Autodesk Fusion 360 part; units mm, degrees
(part 8 of 8)
  spline S32 degree 5 poles (-90.0942, -119.2775) (-90.131, -119.331) (-90.2033, -119.4387) (-90.3076, -119.6028) (-90.4386, -119.8264) (-90.5914, -120.1126) (-90.7364, -120.4035) (-90.8766, -120.6973) (-91.0142, -120.9926) (-91.1501, -121.289) (-91.284, -121.5864) (-91.4155, -121.8852) (-91.5436, -122.1859) (-91.6678, -122.4887) (-91.7881, -122.7937) (-91.9048, -123.1006) (-92.0185, -123.4092) (-92.1295, -123.7191) (-92.2384, -124.0301) (-92.3451, -124.3422) (-92.4496, -124.6553) (-92.5518, -124.9696) (-92.6517, -125.285) (-92.7491, -125.6017) (-92.844, -125.9195) (-92.9366, -126.2385) (-93.027, -126.5585) (-93.1153, -126.8794) (-93.2015, -127.2013) (-93.2857, -127.5241) (-93.368, -127.8478) (-93.4482, -128.1724) (-93.5264, -128.4978) (-93.6027, -128.8241) (-93.6769, -129.1513) (-93.7493, -129.4793) (-93.8197, -129.808) (-93.8882, -130.1376) (-93.9549, -130.4679) (-94.0198, -130.7989) (-94.0829, -131.1307) (-94.1441, -131.4631) (-94.2036, -131.7963) (-94.2613, -132.1301) (-94.3172, -132.4646) (-94.3714, -132.7998) (-94.4239, -133.1356) (-94.4747, -133.4721) (-94.5237, -133.8091) (-94.5711, -134.1468) (-94.6168, -134.4851) (-94.6609, -134.8239) (-94.7033, -135.1634) (-94.744, -135.5033) (-94.7831, -135.8439) (-94.8206, -136.185) (-94.8565, -136.5266) (-94.8908, -136.8687) (-94.9235, -137.2114) (-94.9546, -137.5545) (-94.9842, -137.8982) (-95.0122, -138.2423) (-95.0386, -138.5869) (-95.0635, -138.932) (-95.0869, -139.2775) (-95.1087, -139.6235) (-95.129, -139.97) (-95.1478, -140.3168) (-95.1651, -140.6641) (-95.1808, -141.0118) (-95.1951, -141.36) (-95.2054, -141.6388) (-95.2124, -141.8481) (-95.2168, -141.9877) (-95.2189, -142.0576) knots 0 0 0 0 0 0 0.01428571 0.02857143 0.04285714 0.05714286 0.07142857 0.08571429 0.1 0.11428571 0.12857143 0.14285714 0.15714286 0.17142857 0.18571429 0.2 0.21428571 0.22857143 0.24285714 0.25714286 0.27142857 0.28571429 0.3 0.31428571 0.32857143 0.34285714 0.35714286 0.37142857 0.38571429 0.4 0.41428571 0.42857143 0.44285714 0.45714286 0.47142857 0.48571429 0.5 0.51428571 0.52857143 0.54285714 0.55714286 0.57142857 0.58571429 0.6 0.61428571 0.62857143 0.64285714 0.65714286 0.67142857 0.68571429 0.7 0.71428571 0.72857143 0.74285714 0.75714286 0.77142857 0.78571429 0.8 0.81428571 0.82857143 0.84285714 0.85714286 0.87142857 0.88571429 0.9 0.91428571 0.92857143 0.94285714 0.95714286 0.97142857 0.98571429 1 1 1 1 1 1
  arc A66 (-95.2189, -142.0576) -> (-87.3499, -146.6007) centre (-8.7656, -1.4025) ccw
  spline S33 degree 5 poles (-87.3499, -146.6007) (-87.2904, -146.564) (-87.1717, -146.4904) (-86.9939, -146.3797) (-86.7576, -146.2314) (-86.4632, -146.0449) (-86.17, -145.8574) (-85.8779, -145.6688) (-85.5869, -145.4791) (-85.297, -145.2883) (-85.0083, -145.0964) (-84.7207, -144.9034) (-84.4343, -144.7093) (-84.1491, -144.5141) (-83.865, -144.3178) (-83.5822, -144.1204) (-83.3006, -143.9219) (-83.0202, -143.7222) (-82.7411, -143.5214) (-82.4632, -143.3196) (-82.1865, -143.1165) (-81.9112, -142.9124) (-81.6371, -142.7071) (-81.3644, -142.5007) (-81.0929, -142.2931) (-80.8228, -142.0844) (-80.5541, -141.8745) (-80.2867, -141.6635) (-80.0207, -141.4513) (-79.7561, -141.238) (-79.4929, -141.0235) (-79.2312, -140.8077) (-78.9709, -140.5908) (-78.7122, -140.3728) (-78.4549, -140.1535) (-78.1991, -139.933) (-77.9449, -139.7113) (-77.6922, -139.4884) (-77.441, -139.2642) (-77.1915, -139.0389) (-76.9437, -138.8122) (-76.6975, -138.5844) (-76.453, -138.3552) (-76.2103, -138.1247) (-75.9693, -137.8929) (-75.7301, -137.6599) (-75.4927, -137.4256) (-75.257, -137.1899) (-75.0232, -136.953) (-74.7912, -136.7147) (-74.5613, -136.475) (-74.3336, -136.2339) (-74.108, -135.9912) (-73.8848, -135.747) (-73.6637, -135.5014) (-73.4448, -135.2543) (-73.2279, -135.0058) (-73.0129, -134.7561) (-72.8001, -134.5049) (-72.5897, -134.2522) (-72.3823, -133.9976) (-72.1783, -133.741) (-71.9781, -133.482) (-71.7818, -133.2207) (-71.5887, -132.9575) (-71.3981, -132.6928) (-71.2094, -132.4269) (-71.0224, -132.1601) (-70.8381, -131.8918) (-70.6587, -131.6207) (-70.4873, -131.3453) (-70.3591, -131.1201) (-70.2691, -130.9477) (-70.212, -130.8313) (-70.1841, -130.7726) knots -1 -1 -1 -1 -1 -1 -0.98571429 -0.97142857 -0.95714286 -0.94285714 -0.92857143 -0.91428571 -0.9 -0.88571429 -0.87142857 -0.85714286 -0.84285714 -0.82857143 -0.81428571 -0.8 -0.78571429 -0.77142857 -0.75714286 -0.74285714 -0.72857143 -0.71428571 -0.7 -0.68571429 -0.67142857 -0.65714286 -0.64285714 -0.62857143 -0.61428571 -0.6 -0.58571429 -0.57142857 -0.55714286 -0.54285714 -0.52857143 -0.51428571 -0.5 -0.48571429 -0.47142857 -0.45714286 -0.44285714 -0.42857143 -0.41428571 -0.4 -0.38571429 -0.37142857 -0.35714286 -0.34285714 -0.32857143 -0.31428571 -0.3 -0.28571429 -0.27142857 -0.25714286 -0.24285714 -0.22857143 -0.21428571 -0.2 -0.18571429 -0.17142857 -0.15714286 -0.14285714 -0.12857143 -0.11428571 -0.1 -0.08571429 -0.07142857 -0.05714286 -0.04285714 -0.02857143 -0.01428571 0 0 0 0 0 0
  line L33 (-70.1841, -130.7726) -> (-68.2443, -126.6881)
  arc A67 (-66.146, -125.9273) -> (-68.2443, -126.6881) centre (-66.8103, -127.3691) ccw
  arc A68 (-66.146, -125.9273) -> (-56.2439, -130.0289) centre (-8.7656, -1.4025) ccw
  arc A69 (-55.2981, -132.0506) -> (-56.2439, -130.0289) centre (-56.7937, -131.5181) ccw
  line L34 (-55.2981, -132.0506) -> (-56.8147, -136.3104)
  spline S34 degree 5 poles (-56.8147, -136.3104) (-56.8364, -136.3716) (-56.8784, -136.4943) (-56.9366, -136.6798) (-57.0053, -136.9297) (-57.0788, -137.2457) (-57.1436, -137.5642) (-57.203, -137.8843) (-57.2595, -138.2052) (-57.314, -138.5266) (-57.3664, -138.8486) (-57.416, -139.1712) (-57.4619, -139.4948) (-57.5035, -139.8195) (-57.5408, -140.1452) (-57.5741, -140.4719) (-57.604, -140.7993) (-57.6311, -141.1274) (-57.6557, -141.456) (-57.678, -141.7851) (-57.6979, -142.1146) (-57.7154, -142.4446) (-57.7302, -142.7751) (-57.7423, -143.1062) (-57.7517, -143.4378) (-57.7586, -143.7698) (-57.7631, -144.1023) (-57.7653, -144.4352) (-57.7653, -144.7685) (-57.7631, -145.1021) (-57.7588, -145.436) (-57.7523, -145.7703) (-57.7436, -146.1049) (-57.7328, -146.4398) (-57.7198, -146.775) (-57.7048, -147.1105) (-57.6877, -147.4463) (-57.6686, -147.7824) (-57.6476, -148.1187) (-57.6246, -148.4552) (-57.5996, -148.792) (-57.5728, -149.129) (-57.544, -149.4662) (-57.5133, -149.8036) (-57.4808, -150.1412) (-57.4464, -150.479) (-57.4101, -150.8169) (-57.3721, -151.1551) (-57.3322, -151.4933) (-57.2906, -151.8318) (-57.2472, -152.1703) (-57.202, -152.509) (-57.1551, -152.8479) (-57.1065, -153.1868) (-57.0562, -153.5259) (-57.0041, -153.865) (-56.9504, -154.2043) (-56.8949, -154.5437) (-56.8378, -154.8831) (-56.7791, -155.2226) (-56.7187, -155.5622) (-56.6567, -155.9019) (-56.593, -156.2416) (-56.5277, -156.5813) (-56.4609, -156.9211) (-56.3924, -157.261) (-56.3223, -157.6009) (-56.2507, -157.9408) (-56.1775, -158.2807) (-56.1028, -158.6207) (-56.0265, -158.9606) (-55.9642, -159.2326) (-55.9168, -159.4366) (-55.8849, -159.5726) (-55.8688, -159.6406) knots 0 0 0 0 0 0 0.01428571 0.02857143 0.04285714 0.05714286 0.07142857 0.08571429 0.1 0.11428571 0.12857143 0.14285714 0.15714286 0.17142857 0.18571429 0.2 0.21428571 0.22857143 0.24285714 0.25714286 0.27142857 0.28571429 0.3 0.31428571 0.32857143 0.34285714 0.35714286 0.37142857 0.38571429 0.4 0.41428571 0.42857143 0.44285714 0.45714286 0.47142857 0.48571429 0.5 0.51428571 0.52857143 0.54285714 0.55714286 0.57142857 0.58571429 0.6 0.61428571 0.62857143 0.64285714 0.65714286 0.67142857 0.68571429 0.7 0.71428571 0.72857143 0.74285714 0.75714286 0.77142857 0.78571429 0.8 0.81428571 0.82857143 0.84285714 0.85714286 0.87142857 0.88571429 0.9 0.91428571 0.92857143 0.94285714 0.95714286 0.97142857 0.98571429 1 1 1 1 1 1
  arc A70 (-55.8688, -159.6406) -> (-47.0921, -161.9923) centre (-8.7656, -1.4025) ccw
  spline S35 degree 5 poles (-47.0921, -161.9923) (-47.0442, -161.9414) (-46.9486, -161.8396) (-46.8055, -161.6867) (-46.6156, -161.4823) (-46.3795, -161.226) (-46.1448, -160.969) (-45.9115, -160.7112) (-45.6795, -160.4526) (-45.4489, -160.1933) (-45.2197, -159.9332) (-44.9918, -159.6724) (-44.7654, -159.4108) (-44.5404, -159.1484) (-44.3169, -158.8853) (-44.0948, -158.6214) (-43.8742, -158.3567) (-43.655, -158.0913) (-43.4373, -157.8251) (-43.2211, -157.5582) (-43.0065, -157.2905) (-42.7933, -157.022) (-42.5817, -156.7528) (-42.3717, -156.4828) (-42.1633, -156.2121) (-41.9564, -155.9406) (-41.7511, -155.6683) (-41.5475, -155.3952) (-41.3455, -155.1215) (-41.1451, -154.8469) (-40.9464, -154.5716) (-40.7494, -154.2955) (-40.5542, -154.0186) (-40.3606, -153.741) (-40.1689, -153.4626) (-39.9789, -153.1834) (-39.7907, -152.9034) (-39.6043, -152.6227) (-39.4197, -152.3412) (-39.2371, -152.0589) (-39.0563, -151.7759) (-38.8775, -151.4921) (-38.7006, -151.2074) (-38.5258, -150.922) (-38.3531, -150.6357) (-38.1823, -150.3487) (-38.0136, -150.0609) (-37.847, -149.7723) (-37.6825, -149.4829) (-37.5201, -149.1928) (-37.36, -148.9017) (-37.2024, -148.6098) (-37.0474, -148.3171) (-36.8949, -148.0234) (-36.745, -147.7289) (-36.5975, -147.4336) (-36.4523, -147.1375) (-36.3093, -146.8406) (-36.1687, -146.5429) (-36.0309, -146.2443) (-35.8964, -145.9448) (-35.7659, -145.6441) (-35.6395, -145.3421) (-35.5175, -145.0389) (-35.3991, -144.7347) (-35.2835, -144.4296) (-35.17, -144.124) (-35.0585, -143.8179) (-34.9499, -143.511) (-34.8468, -143.2028) (-34.7525, -142.8924) (-34.687, -142.6416) (-34.6446, -142.4518) (-34.6196, -142.3246) (-34.6079, -142.2607) knots -1 -1 -1 -1 -1 -1 -0.98571429 -0.97142857 -0.95714286 -0.94285714 -0.92857143 -0.91428571 -0.9 -0.88571429 -0.87142857 -0.85714286 -0.84285714 -0.82857143 -0.81428571 -0.8 -0.78571429 -0.77142857 -0.75714286 -0.74285714 -0.72857143 -0.71428571 -0.7 -0.68571429 -0.67142857 -0.65714286 -0.64285714 -0.62857143 -0.61428571 -0.6 -0.58571429 -0.57142857 -0.55714286 -0.54285714 -0.52857143 -0.51428571 -0.5 -0.48571429 -0.47142857 -0.45714286 -0.44285714 -0.42857143 -0.41428571 -0.4 -0.38571429 -0.37142857 -0.35714286 -0.34285714 -0.32857143 -0.31428571 -0.3 -0.28571429 -0.27142857 -0.25714286 -0.24285714 -0.22857143 -0.21428571 -0.2 -0.18571429 -0.17142857 -0.15714286 -0.14285714 -0.12857143 -0.11428571 -0.1 -0.08571429 -0.07142857 -0.05714286 -0.04285714 -0.02857143 -0.01428571 0 0 0 0 0 0
  line L35 (-34.6079, -142.2607) -> (-33.7913, -137.8133)
  arc A71 (-31.9614, -136.5354) -> (-33.7913, -137.8133) centre (-32.2299, -138.1) ccw
  arc A72 (-31.9614, -136.5354) -> (-21.3352, -137.9343) centre (-8.7656, -1.4025) ccw
  arc A73 (-19.8983, -139.6424) -> (-21.3352, -137.9343) centre (-21.4807, -139.5151) ccw
  line L36 (-19.8983, -139.6424) -> (-20.2607, -144.1496)
  spline S36 degree 5 poles (-20.2607, -144.1496) (-20.2659, -144.2143) (-20.2747, -144.3437) (-20.2829, -144.5379) (-20.2845, -144.7971) (-20.2738, -145.1213) (-20.2539, -145.4457) (-20.2284, -145.7703) (-20.1999, -146.0949) (-20.1694, -146.4194) (-20.1367, -146.744) (-20.1011, -147.0685) (-20.0617, -147.3929) (-20.0179, -147.7173) (-19.9696, -148.0416) (-19.9172, -148.3658) (-19.8613, -148.6898) (-19.8026, -149.0137) (-19.7413, -149.3375) (-19.6777, -149.6611) (-19.6116, -149.9846) (-19.5431, -150.3078) (-19.4718, -150.631) (-19.3978, -150.9539) (-19.3211, -151.2766) (-19.2419, -151.5991) (-19.1601, -151.9214) (-19.0761, -152.2436) (-18.9898, -152.5654) (-18.9014, -152.8871) (-18.8107, -153.2085) (-18.718, -153.5297) (-18.623, -153.8507) (-18.5259, -154.1714) (-18.4266, -154.4918) (-18.3252, -154.812) (-18.2218, -155.132) (-18.1164, -155.4516) (-18.009, -155.771) (-17.8997, -156.0902) (-17.7884, -156.409) (-17.6753, -156.7275) (-17.5602, -157.0458) (-17.4432, -157.3638) (-17.3244, -157.6815) (-17.2038, -157.9988) (-17.0813, -158.3159) (-16.957, -158.6326) (-16.831, -158.9491) (-16.7032, -159.2652) (-16.5736, -159.581) (-16.4424, -159.8965) (-16.3094, -160.2116) (-16.1747, -160.5264) (-16.0383, -160.8409) (-15.9002, -161.155) (-15.7605, -161.4688) (-15.6191, -161.7823) (-15.4761, -162.0954) (-15.3315, -162.4081) (-15.1853, -162.7205) (-15.0374, -163.0325) (-14.888, -163.3442) (-14.737, -163.6555) (-14.5845, -163.9664) (-14.4304, -164.277) (-14.2748, -164.5871) (-14.1176, -164.8969) (-13.9589, -165.2063) (-13.7987, -165.5153) (-13.637, -165.824) (-13.5065, -166.0706) (-13.4079, -166.2553) (-13.3419, -166.3784) (-13.3088, -166.44) knots 0 0 0 0 0 0 0.01428571 0.02857143 0.04285714 0.05714286 0.07142857 0.08571429 0.1 0.11428571 0.12857143 0.14285714 0.15714286 0.17142857 0.18571429 0.2 0.21428571 0.22857143 0.24285714 0.25714286 0.27142857 0.28571429 0.3 0.31428571 0.32857143 0.34285714 0.35714286 0.37142857 0.38571429 0.4 0.41428571 0.42857143 0.44285714 0.45714286 0.47142857 0.48571429 0.5 0.51428571 0.52857143 0.54285714 0.55714286 0.57142857 0.58571429 0.6 0.61428571 0.62857143 0.64285714 0.65714286 0.67142857 0.68571429 0.7 0.71428571 0.72857143 0.74285714 0.75714286 0.77142857 0.78571429 0.8 0.81428571 0.82857143 0.84285714 0.85714286 0.87142857 0.88571429 0.9 0.91428571 0.92857143 0.94285714 0.95714286 0.97142857 0.98571429 1 1 1 1 1 1
  arc A74 (-13.3088, -166.44) -> (-4.2224, -166.44) centre (-8.7656, -1.4025) ccw
  spline S37 degree 5 poles (-4.2224, -166.44) (-4.1894, -166.3784) (-4.1233, -166.2553) (-4.0248, -166.0706) (-3.8942, -165.824) (-3.7325, -165.5153) (-3.5723, -165.2063) (-3.4136, -164.8969) (-3.2565, -164.5871) (-3.1008, -164.277) (-2.9468, -163.9664) (-2.7942, -163.6555) (-2.6432, -163.3442) (-2.4938, -163.0325) (-2.346, -162.7205) (-2.1997, -162.4081) (-2.0551, -162.0954) (-1.9121, -161.7823) (-1.7708, -161.4688) (-1.631, -161.155) (-1.493, -160.8409) (-1.3566, -160.5264) (-1.2219, -160.2116) (-1.0889, -159.8965) (-0.9576, -159.581) (-0.828, -159.2652) (-0.7002, -158.9491) (-0.5742, -158.6326) (-0.4499, -158.3159) (-0.3275, -157.9988) (-0.2068, -157.6815) (-0.088, -157.3638) (0.029, -157.0458) (0.144, -156.7275) (0.2572, -156.409) (0.3685, -156.0902) (0.4778, -155.771) (0.5852, -155.4516) (0.6906, -155.132) (0.794, -154.812) (0.8953, -154.4918) (0.9946, -154.1714) (1.0917, -153.8507) (1.1867, -153.5297) (1.2795, -153.2085) (1.3701, -152.8871) (1.4586, -152.5654) (1.5449, -152.2436) (1.6289, -151.9214) (1.7106, -151.5991) (1.7899, -151.2766) (1.8666, -150.9539) (1.9406, -150.631) (2.0118, -150.3078) (2.0804, -149.9846) (2.1464, -149.6611) (2.2101, -149.3375) (2.2713, -149.0137) (2.3301, -148.6898) (2.386, -148.3658) (2.4383, -148.0416) (2.4866, -147.7173) (2.5305, -147.3929) (2.5699, -147.0685) (2.6055, -146.744) (2.6382, -146.4194) (2.6687, -146.0949) (2.6972, -145.7703) (2.7227, -145.4457) (2.7425, -145.1213) (2.7533, -144.7971) (2.7516, -144.5379) (2.7434, -144.3437) (2.7347, -144.2143) (2.7295, -144.1496) knots -1 -1 -1 -1 -1 -1 -0.98571429 -0.97142857 -0.95714286 -0.94285714 -0.92857143 -0.91428571 -0.9 -0.88571429 -0.87142857 -0.85714286 -0.84285714 -0.82857143 -0.81428571 -0.8 -0.78571429 -0.77142857 -0.75714286 -0.74285714 -0.72857143 -0.71428571 -0.7 -0.68571429 -0.67142857 -0.65714286 -0.64285714 -0.62857143 -0.61428571 -0.6 -0.58571429 -0.57142857 -0.55714286 -0.54285714 -0.52857143 -0.51428571 -0.5 -0.48571429 -0.47142857 -0.45714286 -0.44285714 -0.42857143 -0.41428571 -0.4 -0.38571429 -0.37142857 -0.35714286 -0.34285714 -0.32857143 -0.31428571 -0.3 -0.28571429 -0.27142857 -0.25714286 -0.24285714 -0.22857143 -0.21428571 -0.2 -0.18571429 -0.17142857 -0.15714286 -0.14285714 -0.12857143 -0.11428571 -0.1 -0.08571429 -0.07142857 -0.05714286 -0.04285714 -0.02857143 -0.01428571 0 0 0 0 0 0
  line L37 (2.7295, -144.1496) -> (2.3671, -139.6424)
  arc A75 (3.804, -137.9343) -> (2.3671, -139.6424) centre (3.9495, -139.5151) ccw
  arc A76 (3.804, -137.9343) -> (14.4301, -136.5354) centre (-8.7656, -1.4025) ccw
  arc A77 (16.2601, -137.8133) -> (14.4301, -136.5354) centre (14.6987, -138.1) ccw
  line L38 (16.2601, -137.8133) -> (17.0766, -142.2607)
  spline S38 degree 5 poles (17.0766, -142.2607) (17.0884, -142.3246) (17.1134, -142.4518) (17.1557, -142.6416) (17.2212, -142.8924) (17.3155, -143.2028) (17.4187, -143.511) (17.5273, -143.8179) (17.6388, -144.124) (17.7523, -144.4296) (17.8679, -144.7347) (17.9862, -145.0389) (18.1083, -145.3421) (18.2346, -145.6441) (18.3652, -145.9448) (18.4997, -146.2443) (18.6375, -146.5429) (18.7781, -146.8406) (18.9211, -147.1375) (19.0663, -147.4336) (19.2138, -147.7289) (19.3637, -148.0234) (19.5162, -148.3171) (19.6712, -148.6098) (19.8288, -148.9017) (19.9889, -149.1928) (20.1512, -149.4829) (20.3158, -149.7723) (20.4824, -150.0609) (20.6511, -150.3487) (20.8218, -150.6357) (20.9946, -150.922) (21.1694, -151.2074) (21.3462, -151.4921) (21.525, -151.7759) (21.7058, -152.0589) (21.8885, -152.3412) (22.0731, -152.6227) (22.2594, -152.9034) (22.4476, -153.1834) (22.6376, -153.4626) (22.8294, -153.741) (23.0229, -154.0186) (23.2182, -154.2955) (23.4152, -154.5716) (23.6139, -154.8469) (23.8142, -155.1215) (24.0162, -155.3952) (24.2199, -155.6683) (24.4251, -155.9406) (24.632, -156.2121) (24.8405, -156.4828) (25.0505, -156.7528) (25.2621, -157.022) (25.4752, -157.2905) (25.6899, -157.5582) (25.9061, -157.8251) (26.1238, -158.0913) (26.3429, -158.3567) (26.5636, -158.6214) (26.7857, -158.8853) (27.0092, -159.1484) (27.2342, -159.4108) (27.4606, -159.6724) (27.6884, -159.9332) (27.9176, -160.1933) (28.1483, -160.4526) (28.3802, -160.7112) (28.6136, -160.969) (28.8483, -161.226) (29.0844, -161.4823) (29.2743, -161.6867) (29.4173, -161.8396) (29.513, -161.9414) (29.5609, -161.9923) knots 0 0 0 0 0 0 0.01428571 0.02857143 0.04285714 0.05714286 0.07142857 0.08571429 0.1 0.11428571 0.12857143 0.14285714 0.15714286 0.17142857 0.18571429 0.2 0.21428571 0.22857143 0.24285714 0.25714286 0.27142857 0.28571429 0.3 0.31428571 0.32857143 0.34285714 0.35714286 0.37142857 0.38571429 0.4 0.41428571 0.42857143 0.44285714 0.45714286 0.47142857 0.48571429 0.5 0.51428571 0.52857143 0.54285714 0.55714286 0.57142857 0.58571429 0.6 0.61428571 0.62857143 0.64285714 0.65714286 0.67142857 0.68571429 0.7 0.71428571 0.72857143 0.74285714 0.75714286 0.77142857 0.78571429 0.8 0.81428571 0.82857143 0.84285714 0.85714286 0.87142857 0.88571429 0.9 0.91428571 0.92857143 0.94285714 0.95714286 0.97142857 0.98571429 1 1 1 1 1 1
  arc A78 (29.5609, -161.9923) -> (38.3376, -159.6406) centre (-8.7656, -1.4025) ccw
  spline S39 degree 5 poles (38.3376, -159.6406) (38.3536, -159.5726) (38.3855, -159.4366) (38.4329, -159.2326) (38.4952, -158.9606) (38.5715, -158.6207) (38.6463, -158.2807) (38.7195, -157.9408) (38.7911, -157.6009) (38.8611, -157.261) (38.9296, -156.9211) (38.9965, -156.5813) (39.0618, -156.2416) (39.1254, -155.9019) (39.1875, -155.5622) (39.2478, -155.2226) (39.3066, -154.8831) (39.3637, -154.5437) (39.4191, -154.2043) (39.4729, -153.865) (39.5249, -153.5259) (39.5753, -153.1868) (39.6239, -152.8479) (39.6708, -152.509) (39.716, -152.1703) (39.7594, -151.8318) (39.801, -151.4933) (39.8408, -151.1551) (39.8789, -150.8169) (39.9151, -150.479) (39.9495, -150.1412) (39.9821, -149.8036) (40.0127, -149.4662) (40.0415, -149.129) (40.0684, -148.792) (40.0933, -148.4552) (40.1163, -148.1187) (40.1374, -147.7824) (40.1565, -147.4463) (40.1736, -147.1105) (40.1886, -146.775) (40.2015, -146.4398) (40.2124, -146.1049) (40.221, -145.7703) (40.2275, -145.436) (40.2319, -145.1021) (40.2341, -144.7685) (40.2341, -144.4352) (40.2319, -144.1023) (40.2274, -143.7698) (40.2205, -143.4378) (40.211, -143.1062) (40.1989, -142.7751) (40.1841, -142.4446) (40.1667, -142.1146) (40.1468, -141.7851) (40.1245, -141.456) (40.0999, -141.1274) (40.0728, -140.7993) (40.0429, -140.4719) (40.0095, -140.1452) (39.9723, -139.8195) (39.9307, -139.4948) (39.8848, -139.1712) (39.8352, -138.8486) (39.7827, -138.5266) (39.7282, -138.2052) (39.6717, -137.8843) (39.6123, -137.5642) (39.5476, -137.2457) (39.474, -136.9297) (39.4054, -136.6798) (39.3472, -136.4943) (39.3052, -136.3716) (39.2834, -136.3104) knots -1 -1 -1 -1 -1 -1 -0.98571429 -0.97142857 -0.95714286 -0.94285714 -0.92857143 -0.91428571 -0.9 -0.88571429 -0.87142857 -0.85714286 -0.84285714 -0.82857143 -0.81428571 -0.8 -0.78571429 -0.77142857 -0.75714286 -0.74285714 -0.72857143 -0.71428571 -0.7 -0.68571429 -0.67142857 -0.65714286 -0.64285714 -0.62857143 -0.61428571 -0.6 -0.58571429 -0.57142857 -0.55714286 -0.54285714 -0.52857143 -0.51428571 -0.5 -0.48571429 -0.47142857 -0.45714286 -0.44285714 -0.42857143 -0.41428571 -0.4 -0.38571429 -0.37142857 -0.35714286 -0.34285714 -0.32857143 -0.31428571 -0.3 -0.28571429 -0.27142857 -0.25714286 -0.24285714 -0.22857143 -0.21428571 -0.2 -0.18571429 -0.17142857 -0.15714286 -0.14285714 -0.12857143 -0.11428571 -0.1 -0.08571429 -0.07142857 -0.05714286 -0.04285714 -0.02857143 -0.01428571 0 0 0 0 0 0
  line L39 (39.2834, -136.3104) -> (37.7669, -132.0506)
  arc A79 (38.7127, -130.0289) -> (37.7669, -132.0506) centre (39.2624, -131.5181) ccw
  arc A80 (38.7127, -130.0289) -> (48.6147, -125.9273) centre (-8.7656, -1.4025) ccw
  arc A81 (50.7131, -126.6881) -> (48.6147, -125.9273) centre (49.2791, -127.3691) ccw
  line L40 (50.7131, -126.6881) -> (52.6529, -130.7726)
  spline S40 degree 5 poles (52.6529, -130.7726) (52.6807, -130.8313) (52.7378, -130.9477) (52.8278, -131.1201) (52.956, -131.3453) (53.1274, -131.6207) (53.3069, -131.8918) (53.4912, -132.1601) (53.6781, -132.4269) (53.8669, -132.6928) (54.0575, -132.9575) (54.2505, -133.2207) (54.4469, -133.482) (54.6471, -133.741) (54.851, -133.9976) (55.0585, -134.2522) (55.2689, -134.5049) (55.4817, -134.7561) (55.6966, -135.0058) (55.9136, -135.2543) (56.1325, -135.5014) (56.3535, -135.747) (56.5768, -135.9912) (56.8023, -136.2339) (57.0301, -136.475) (57.26, -136.7147) (57.4919, -136.953) (57.7258, -137.1899) (57.9614, -137.4256) (58.1989, -137.6599) (58.4381, -137.8929) (58.679, -138.1247) (58.9217, -138.3552) (59.1662, -138.5844) (59.4124, -138.8122) (59.6603, -139.0389) (59.9098, -139.2642) (60.1609, -139.4884) (60.4136, -139.7113) (60.6679, -139.933) (60.9236, -140.1535) (61.1809, -140.3728) (61.4397, -140.5908) (61.7, -140.8077) (61.9617, -141.0235) (62.2249, -141.238) (62.4895, -141.4513) (62.7555, -141.6635) (63.0228, -141.8745) (63.2916, -142.0844) (63.5617, -142.2931) (63.8331, -142.5007) (64.1059, -142.7071) (64.3799, -142.9124) (64.6553, -143.1165) (64.9319, -143.3196) (65.2098, -143.5214) (65.489, -143.7222) (65.7694, -143.9219) (66.051, -144.1204) (66.3338, -144.3178) (66.6178, -144.5141) (66.9031, -144.7093) (67.1895, -144.9034) (67.477, -145.0964) (67.7658, -145.2883) (68.0556, -145.4791) (68.3466, -145.6688) (68.6388, -145.8574) (68.932, -146.0449) (69.2263, -146.2314) (69.4627, -146.3797) (69.6405, -146.4904) (69.7592, -146.564) (69.8186, -146.6007) knots 0 0 0 0 0 0 0.01428571 0.02857143 0.04285714 0.05714286 0.07142857 0.08571429 0.1 0.11428571 0.12857143 0.14285714 0.15714286 0.17142857 0.18571429 0.2 0.21428571 0.22857143 0.24285714 0.25714286 0.27142857 0.28571429 0.3 0.31428571 0.32857143 0.34285714 0.35714286 0.37142857 0.38571429 0.4 0.41428571 0.42857143 0.44285714 0.45714286 0.47142857 0.48571429 0.5 0.51428571 0.52857143 0.54285714 0.55714286 0.57142857 0.58571429 0.6 0.61428571 0.62857143 0.64285714 0.65714286 0.67142857 0.68571429 0.7 0.71428571 0.72857143 0.74285714 0.75714286 0.77142857 0.78571429 0.8 0.81428571 0.82857143 0.84285714 0.85714286 0.87142857 0.88571429 0.9 0.91428571 0.92857143 0.94285714 0.95714286 0.97142857 0.98571429 1 1 1 1 1 1
  arc A82 (69.8186, -146.6007) -> (77.6876, -142.0576) centre (-8.7656, -1.4025) ccw
  spline S41 degree 5 poles (77.6876, -142.0576) (77.6855, -141.9877) (77.6811, -141.8481) (77.6741, -141.6388) (77.6639, -141.36) (77.6496, -141.0118) (77.6338, -140.6641) (77.6165, -140.3168) (77.5977, -139.97) (77.5774, -139.6235) (77.5556, -139.2775) (77.5323, -138.932) (77.5074, -138.5869) (77.4809, -138.2423) (77.453, -137.8982) (77.4234, -137.5545) (77.3923, -137.2114) (77.3596, -136.8687) (77.3253, -136.5266) (77.2894, -136.185) (77.2519, -135.8439) (77.2128, -135.5033) (77.172, -135.1634) (77.1296, -134.8239) (77.0856, -134.4851) (77.0399, -134.1468) (76.9925, -133.8091) (76.9434, -133.4721) (76.8927, -133.1356) (76.8402, -132.7998) (76.786, -132.4646) (76.7301, -132.1301) (76.6724, -131.7963) (76.6129, -131.4631) (76.5516, -131.1307) (76.4886, -130.7989) (76.4237, -130.4679) (76.357, -130.1376) (76.2884, -129.808) (76.218, -129.4793) (76.1457, -129.1513) (76.0714, -128.8241) (75.9952, -128.4978) (75.917, -128.1724) (75.8367, -127.8478) (75.7545, -127.5241) (75.6703, -127.2013) (75.584, -126.8794) (75.4958, -126.5585) (75.4054, -126.2385) (75.3128, -125.9195) (75.2178, -125.6017) (75.1204, -125.285) (75.0206, -124.9696) (74.9183, -124.6553) (74.8138, -124.3422) (74.7071, -124.0301) (74.5983, -123.7191) (74.4872, -123.4092) (74.3736, -123.1006) (74.2568, -122.7937) (74.1365, -122.4887) (74.0123, -122.1859) (73.8842, -121.8852) (73.7528, -121.5864) (73.6188, -121.289) (73.483, -120.9926) (73.3454, -120.6973) (73.2052, -120.4035) (73.0602, -120.1126) (72.9073, -119.8264) (72.7763, -119.6028) (72.6721, -119.4387) (72.5998, -119.331) (72.5629, -119.2775) knots -1 -1 -1 -1 -1 -1 -0.98571429 -0.97142857 -0.95714286 -0.94285714 -0.92857143 -0.91428571 -0.9 -0.88571429 -0.87142857 -0.85714286 -0.84285714 -0.82857143 -0.81428571 -0.8 -0.78571429 -0.77142857 -0.75714286 -0.74285714 -0.72857143 -0.71428571 -0.7 -0.68571429 -0.67142857 -0.65714286 -0.64285714 -0.62857143 -0.61428571 -0.6 -0.58571429 -0.57142857 -0.55714286 -0.54285714 -0.52857143 -0.51428571 -0.5 -0.48571429 -0.47142857 -0.45714286 -0.44285714 -0.42857143 -0.41428571 -0.4 -0.38571429 -0.37142857 -0.35714286 -0.34285714 -0.32857143 -0.31428571 -0.3 -0.28571429 -0.27142857 -0.25714286 -0.24285714 -0.22857143 -0.21428571 -0.2 -0.18571429 -0.17142857 -0.15714286 -0.14285714 -0.12857143 -0.11428571 -0.1 -0.08571429 -0.07142857 -0.05714286 -0.04285714 -0.02857143 -0.01428571 0 0 0 0 0 0
  line L41 (72.5629, -119.2775) -> (69.9955, -115.5554)
  arc A83 (70.3859, -113.3577) -> (69.9955, -115.5554) centre (71.3023, -114.654) ccw
  arc A84 (70.3859, -113.3577) -> (78.8889, -106.8331) centre (-8.7656, -1.4025) ccw
  arc A85 (81.1127, -107.0249) -> (78.8889, -106.8331) centre (79.9038, -108.0538) ccw
  line L42 (81.1127, -107.0249) -> (84.0435, -110.4682)
  spline S42 degree 5 poles (84.0435, -110.4682) (84.0856, -110.5176) (84.1709, -110.6153) (84.3025, -110.7585) (84.4846, -110.9429) (84.7214, -111.1646) (84.9649, -111.3799) (85.2124, -111.5914) (85.462, -111.8007) (85.7131, -112.0087) (85.9658, -112.215) (86.2204, -112.4193) (86.4777, -112.6209) (86.738, -112.8192) (87.0015, -113.0144) (87.2677, -113.2066) (87.5364, -113.3962) (87.807, -113.5837) (88.0792, -113.7693) (88.353, -113.9532) (88.6285, -114.1352) (88.9056, -114.3153) (89.1844, -114.4934) (89.4651, -114.6694) (89.7475, -114.8434) (90.0316, -115.0154) (90.3173, -115.1855) (90.6045, -115.3538) (90.8931, -115.5204) (91.1831, -115.6854) (91.4745, -115.8486) (91.7672, -116.0101) (92.0613, -116.1699) (92.3568, -116.3279) (92.6536, -116.4843) (92.9516, -116.6391) (93.251, -116.7922) (93.5516, -116.9437) (93.8533, -117.0936) (94.1563, -117.242) (94.4604, -117.3887) (94.7657, -117.534) (95.0721, -117.6776) (95.3797, -117.8198) (95.6883, -117.9604) (95.998, -118.0995) (96.3088, -118.2371) (96.6207, -118.3732) (96.9335, -118.5078) (97.2475, -118.641) (97.5624, -118.7727) (97.8783, -118.9029) (98.1952, -119.0317) (98.513, -119.1591) (98.8318, -119.285) (99.1516, -119.4095) (99.4723, -119.5326) (99.7939, -119.6543) (100.1164, -119.7746) (100.4398, -119.8934) (100.7641, -120.0109) (101.0892, -120.127) (101.4153, -120.2418) (101.7421, -120.3551) (102.0699, -120.4671) (102.3984, -120.5777) (102.7278, -120.687) (103.058, -120.7949) (103.389, -120.9015) (103.7207, -121.0068) (104.0533, -121.1107) (104.32, -121.1927) (104.5204, -121.2537) (104.6541, -121.294) (104.721, -121.3141) knots 0 0 0 0 0 0 0.01428571 0.02857143 0.04285714 0.05714286 0.07142857 0.08571429 0.1 0.11428571 0.12857143 0.14285714 0.15714286 0.17142857 0.18571429 0.2 0.21428571 0.22857143 0.24285714 0.25714286 0.27142857 0.28571429 0.3 0.31428571 0.32857143 0.34285714 0.35714286 0.37142857 0.38571429 0.4 0.41428571 0.42857143 0.44285714 0.45714286 0.47142857 0.48571429 0.5 0.51428571 0.52857143 0.54285714 0.55714286 0.57142857 0.58571429 0.6 0.61428571 0.62857143 0.64285714 0.65714286 0.67142857 0.68571429 0.7 0.71428571 0.72857143 0.74285714 0.75714286 0.77142857 0.78571429 0.8 0.81428571 0.82857143 0.84285714 0.85714286 0.87142857 0.88571429 0.9 0.91428571 0.92857143 0.94285714 0.95714286 0.97142857 0.98571429 1 1 1 1 1 1
  arc A86 (104.721, -121.3141) -> (111.146, -114.8891) centre (-8.7656, -1.4025) ccw
  spline S43 degree 5 poles (111.146, -114.8891) (111.1259, -114.8222) (111.0855, -114.6885) (111.0246, -114.4881) (110.9425, -114.2214) (110.8386, -113.8889) (110.7334, -113.5571) (110.6268, -113.2261) (110.5189, -112.8959) (110.4096, -112.5665) (110.299, -112.238) (110.187, -111.9103) (110.0736, -111.5834) (109.9589, -111.2573) (109.8428, -110.9322) (109.7253, -110.6079) (109.6064, -110.2845) (109.4862, -109.962) (109.3645, -109.6404) (109.2414, -109.3197) (109.1169, -108.9999) (108.991, -108.6811) (108.8636, -108.3633) (108.7348, -108.0464) (108.6046, -107.7305) (108.4729, -107.4156) (108.3397, -107.1017) (108.2051, -106.7888) (108.069, -106.4769) (107.9314, -106.1661) (107.7923, -105.8564) (107.6517, -105.5478) (107.5095, -105.2402) (107.3658, -104.9338) (107.2206, -104.6285) (107.0738, -104.3244) (106.9255, -104.0215) (106.7756, -103.7197) (106.6241, -103.4191) (106.471, -103.1198) (106.3162, -102.8217) (106.1598, -102.5249) (106.0017, -102.2294) (105.8419, -101.9353) (105.6804, -101.6426) (105.5172, -101.3512) (105.3523, -101.0612) (105.1857, -100.7726) (105.0174, -100.4854) (104.8473, -100.1997) (104.6752, -99.9156) (104.5013, -99.6332) (104.3252, -99.3525) (104.1472, -99.0737) (103.9671, -98.7966) (103.785, -98.5212) (103.6012, -98.2473) (103.4156, -97.9751) (103.2281, -97.7045) (103.0385, -97.4359) (102.8463, -97.1696) (102.6511, -96.9062) (102.4528, -96.6458) (102.2512, -96.3885) (102.0469, -96.1339) (101.8405, -95.8813) (101.6326, -95.6302) (101.4232, -95.3805) (101.2118, -95.133) (100.9964, -94.8896) (100.7748, -94.6527) (100.5904, -94.4706) (100.4472, -94.3391) (100.3495, -94.2537) (100.3, -94.2117) knots -1 -1 -1 -1 -1 -1 -0.98571429 -0.97142857 -0.95714286 -0.94285714 -0.92857143 -0.91428571 -0.9 -0.88571429 -0.87142857 -0.85714286 -0.84285714 -0.82857143 -0.81428571 -0.8 -0.78571429 -0.77142857 -0.75714286 -0.74285714 -0.72857143 -0.71428571 -0.7 -0.68571429 -0.67142857 -0.65714286 -0.64285714 -0.62857143 -0.61428571 -0.6 -0.58571429 -0.57142857 -0.55714286 -0.54285714 -0.52857143 -0.51428571 -0.5 -0.48571429 -0.47142857 -0.45714286 -0.44285714 -0.42857143 -0.41428571 -0.4 -0.38571429 -0.37142857 -0.35714286 -0.34285714 -0.32857143 -0.31428571 -0.3 -0.28571429 -0.27142857 -0.25714286 -0.24285714 -0.22857143 -0.21428571 -0.2 -0.18571429 -0.17142857 -0.15714286 -0.14285714 -0.12857143 -0.11428571 -0.1 -0.08571429 -0.07142857 -0.05714286 -0.04285714 -0.02857143 -0.01428571 0 0 0 0 0 0
  line L43 (100.3, -94.2117) -> (96.8567, -91.2808)
  arc A87 (96.665, -89.057) -> (96.8567, -91.2808) centre (97.8857, -90.0719) ccw
  arc A88 (96.665, -89.057) -> (103.1896, -80.554) centre (-8.7656, -1.4025) ccw
  arc A89 (105.3872, -80.1636) -> (103.1896, -80.554) centre (104.4859, -81.4704) ccw
  line L44 (105.3872, -80.1636) -> (109.1094, -82.7311)
  spline S44 degree 5 poles (109.1094, -82.7311) (109.1629, -82.7679) (109.2706, -82.8402) (109.4347, -82.9445) (109.6583, -83.0754) (109.9445, -83.2283) (110.2354, -83.3733) (110.5291, -83.5135) (110.8245, -83.6511) (111.1208, -83.7869) (111.4183, -83.9209) (111.7171, -84.0524) (112.0178, -84.1804) (112.3206, -84.3046) (112.6256, -84.4249) (112.9325, -84.5417) (113.2411, -84.6553) (113.551, -84.7664) (113.862, -84.8752) (114.1741, -84.9819) (114.4872, -85.0865) (114.8015, -85.1887) (115.1169, -85.2886) (115.4336, -85.3859) (115.7514, -85.4809) (116.0704, -85.5735) (116.3904, -85.6639) (116.7113, -85.7522) (117.0332, -85.8384) (117.356, -85.9226) (117.6797, -86.0049) (118.0043, -86.0851) (118.3297, -86.1633) (118.656, -86.2396) (118.9832, -86.3138) (119.3111, -86.3861) (119.6399, -86.4566) (119.9695, -86.5251) (120.2998, -86.5918) (120.6308, -86.6567) (120.9625, -86.7197) (121.295, -86.781) (121.6282, -86.8405) (121.962, -86.8982) (122.2965, -86.9541) (122.6317, -87.0083) (122.9675, -87.0608) (123.304, -87.1116) (123.641, -87.1606) (123.9787, -87.208) (124.317, -87.2537) (124.6558, -87.2977) (124.9952, -87.3401) (125.3352, -87.3809) (125.6758, -87.42) (126.0169, -87.4575) (126.3585, -87.4934) (126.7006, -87.5277) (127.0432, -87.5604) (127.3864, -87.5915) (127.73, -87.6211) (128.0742, -87.6491) (128.4188, -87.6755) (128.7639, -87.7004) (129.1094, -87.7237) (129.4554, -87.7456) (129.8019, -87.7659) (130.1487, -87.7847) (130.496, -87.8019) (130.8437, -87.8177) (131.1918, -87.832) (131.4707, -87.8422) (131.68, -87.8493) (131.8196, -87.8536) (131.8894, -87.8557) knots 0 0 0 0 0 0 0.01428571 0.02857143 0.04285714 0.05714286 0.07142857 0.08571429 0.1 0.11428571 0.12857143 0.14285714 0.15714286 0.17142857 0.18571429 0.2 0.21428571 0.22857143 0.24285714 0.25714286 0.27142857 0.28571429 0.3 0.31428571 0.32857143 0.34285714 0.35714286 0.37142857 0.38571429 0.4 0.41428571 0.42857143 0.44285714 0.45714286 0.47142857 0.48571429 0.5 0.51428571 0.52857143 0.54285714 0.55714286 0.57142857 0.58571429 0.6 0.61428571 0.62857143 0.64285714 0.65714286 0.67142857 0.68571429 0.7 0.71428571 0.72857143 0.74285714 0.75714286 0.77142857 0.78571429 0.8 0.81428571 0.82857143 0.84285714 0.85714286 0.87142857 0.88571429 0.9 0.91428571 0.92857143 0.94285714 0.95714286 0.97142857 0.98571429 1 1 1 1 1 1
  arc A90 (131.8894, -87.8557) -> (136.4326, -79.9867) centre (-8.7656, -1.4025) ccw
  spline S45 degree 5 poles (136.4326, -79.9867) (136.3959, -79.9273) (136.3223, -79.8086) (136.2115, -79.6308) (136.0633, -79.3945) (135.8768, -79.1001) (135.6893, -78.8069) (135.5007, -78.5148) (135.311, -78.2238) (135.1202, -77.9339) (134.9283, -77.6452) (134.7353, -77.3576) (134.5412, -77.0712) (134.346, -76.786) (134.1497, -76.5019) (133.9523, -76.2191) (133.7537, -75.9375) (133.5541, -75.6571) (133.3533, -75.3779) (133.1514, -75.1) (132.9484, -74.8234) (132.7443, -74.548) (132.539, -74.274) (132.3326, -74.0012) (132.125, -73.7298) (131.9163, -73.4597) (131.7064, -73.191) (131.4954, -72.9236) (131.2832, -72.6576) (131.0699, -72.393) (130.8553, -72.1298) (130.6396, -71.8681) (130.4227, -71.6078) (130.2046, -71.349) (129.9854, -71.0918) (129.7649, -70.836) (129.5432, -70.5817) (129.3202, -70.329) (129.0961, -70.0779) (128.8707, -69.8284) (128.6441, -69.5805) (128.4162, -69.3343) (128.1871, -69.0899) (127.9566, -68.8471) (127.7248, -68.6062) (127.4918, -68.367) (127.2574, -68.1295) (127.0218, -67.8939) (126.7849, -67.6601) (126.5466, -67.4281) (126.3069, -67.1982) (126.0658, -66.9704) (125.8231, -66.7449) (125.5789, -66.5216) (125.3332, -66.3006) (125.0861, -66.0817) (124.8377, -65.8648) (124.5879, -65.6498) (124.3368, -65.437) (124.0841, -65.2266) (123.8295, -65.0191) (123.5728, -64.8152) (123.3139, -64.615) (123.0526, -64.4187) (122.7894, -64.2256) (122.5246, -64.035) (122.2588, -63.8463) (121.992, -63.6593) (121.7236, -63.475) (121.4526, -63.2956) (121.1772, -63.1242) (120.9519, -62.996) (120.7796, -62.906) (120.6631, -62.8488) (120.6045, -62.821) knots -1 -1 -1 -1 -1 -1 -0.98571429 -0.97142857 -0.95714286 -0.94285714 -0.92857143 -0.91428571 -0.9 -0.88571429 -0.87142857 -0.85714286 -0.84285714 -0.82857143 -0.81428571 -0.8 -0.78571429 -0.77142857 -0.75714286 -0.74285714 -0.72857143 -0.71428571 -0.7 -0.68571429 -0.67142857 -0.65714286 -0.64285714 -0.62857143 -0.61428571 -0.6 -0.58571429 -0.57142857 -0.55714286 -0.54285714 -0.52857143 -0.51428571 -0.5 -0.48571429 -0.47142857 -0.45714286 -0.44285714 -0.42857143 -0.41428571 -0.4 -0.38571429 -0.37142857 -0.35714286 -0.34285714 -0.32857143 -0.31428571 -0.3 -0.28571429 -0.27142857 -0.25714286 -0.24285714 -0.22857143 -0.21428571 -0.2 -0.18571429 -0.17142857 -0.15714286 -0.14285714 -0.12857143 -0.11428571 -0.1 -0.08571429 -0.07142857 -0.05714286 -0.04285714 -0.02857143 -0.01428571 0 0 0 0 0 0
  line L45 (120.6045, -62.821) -> (116.52, -60.8812)
  arc A91 (115.7592, -58.7828) -> (116.52, -60.8812) centre (117.201, -59.4472) ccw
  arc A92 (115.7592, -58.7828) -> (119.8607, -48.8808) centre (-8.7656, -1.4025) ccw
  arc A93 (121.8825, -47.935) -> (119.8607, -48.8808) centre (121.35, -49.4305) ccw
  line L46 (121.8825, -47.935) -> (126.1423, -49.4516)
  spline S46 degree 5 poles (126.1423, -49.4516) (126.2035, -49.4733) (126.3262, -49.5153) (126.5117, -49.5735) (126.7616, -49.6421) (127.0776, -49.7157) (127.3961, -49.7805) (127.7162, -49.8399) (128.037, -49.8963) (128.3585, -49.9509) (128.6804, -50.0033) (129.0031, -50.0529) (129.3267, -50.0988) (129.6513, -50.1404) (129.9771, -50.1777) (130.3037, -50.211) (130.6312, -50.2409) (130.9593, -50.268) (131.2879, -50.2926) (131.6169, -50.3149) (131.9465, -50.3348) (132.2765, -50.3523) (132.607, -50.3671) (132.9381, -50.3792) (133.2697, -50.3886) (133.6017, -50.3955) (133.9342, -50.4) (134.2671, -50.4022) (134.6004, -50.4022) (134.9339, -50.4) (135.2679, -50.3956) (135.6022, -50.3891) (135.9367, -50.3805) (136.2717, -50.3697) (136.6069, -50.3567) (136.9424, -50.3417) (137.2782, -50.3246) (137.6143, -50.3055) (137.9506, -50.2845) (138.2871, -50.2615) (138.6239, -50.2365) (138.9609, -50.2096) (139.2981, -50.1809) (139.6355, -50.1502) (139.9731, -50.1176) (140.3109, -50.0832) (140.6488, -50.047) (140.9869, -50.009) (141.3252, -49.9691) (141.6636, -49.9275) (142.0022, -49.8841) (142.3409, -49.8389) (142.6797, -49.792) (143.0187, -49.7434) (143.3578, -49.693) (143.6969, -49.641) (144.0362, -49.5872) (144.3755, -49.5318) (144.715, -49.4747) (145.0545, -49.416) (145.3941, -49.3556) (145.7337, -49.2935) (146.0734, -49.2299) (146.4132, -49.1646) (146.753, -49.0977) (147.0929, -49.0293) (147.4328, -48.9592) (147.7727, -48.8876) (148.1126, -48.8144) (148.4525, -48.7396) (148.7925, -48.6633) (149.0645, -48.6011) (149.2685, -48.5537) (149.4045, -48.5217) (149.4725, -48.5057) knots 0 0 0 0 0 0 0.01428571 0.02857143 0.04285714 0.05714286 0.07142857 0.08571429 0.1 0.11428571 0.12857143 0.14285714 0.15714286 0.17142857 0.18571429 0.2 0.21428571 0.22857143 0.24285714 0.25714286 0.27142857 0.28571429 0.3 0.31428571 0.32857143 0.34285714 0.35714286 0.37142857 0.38571429 0.4 0.41428571 0.42857143 0.44285714 0.45714286 0.47142857 0.48571429 0.5 0.51428571 0.52857143 0.54285714 0.55714286 0.57142857 0.58571429 0.6 0.61428571 0.62857143 0.64285714 0.65714286 0.67142857 0.68571429 0.7 0.71428571 0.72857143 0.74285714 0.75714286 0.77142857 0.78571429 0.8 0.81428571 0.82857143 0.84285714 0.85714286 0.87142857 0.88571429 0.9 0.91428571 0.92857143 0.94285714 0.95714286 0.97142857 0.98571429 1 1 1 1 1 1
  arc A94 (149.4725, -48.5057) -> (151.8242, -39.729) centre (-8.7656, -1.4025) ccw
  spline S47 degree 5 poles (151.8242, -39.729) (151.7733, -39.6811) (151.6715, -39.5855) (151.5185, -39.4424) (151.3141, -39.2525) (151.0579, -39.0164) (150.8009, -38.7817) (150.5431, -38.5484) (150.2845, -38.3164) (150.0252, -38.0858) (149.7651, -37.8565) (149.5042, -37.6287) (149.2426, -37.4023) (148.9803, -37.1773) (148.7171, -36.9538) (148.4532, -36.7317) (148.1886, -36.511) (147.9232, -36.2919) (147.657, -36.0742) (147.3901, -35.858) (147.1224, -35.6434) (146.8539, -35.4302) (146.5847, -35.2186) (146.3147, -35.0086) (146.0439, -34.8001) (145.7724, -34.5933) (145.5002, -34.388) (145.2271, -34.1843) (144.9533, -33.9823) (144.6788, -33.782) (144.4034, -33.5833) (144.1273, -33.3863) (143.8505, -33.191) (143.5728, -32.9975) (143.2944, -32.8058) (143.0153, -32.6158) (142.7353, -32.4276) (142.4546, -32.2412) (142.1731, -32.0566) (141.8908, -31.8739) (141.6078, -31.6932) (141.3239, -31.5143) (141.0393, -31.3375) (140.7539, -31.1627) (140.4676, -30.9899) (140.1806, -30.8192) (139.8928, -30.6505) (139.6042, -30.4839) (139.3148, -30.3193) (139.0246, -30.157) (138.7336, -29.9969) (138.4417, -29.8393) (138.149, -29.6843) (137.8553, -29.5318) (137.5608, -29.3819) (137.2655, -29.2344) (136.9693, -29.0892) (136.6724, -28.9462) (136.3748, -28.8056) (136.0762, -28.6678) (135.7767, -28.5333) (135.4759, -28.4027) (135.174, -28.2764) (134.8708, -28.1544) (134.5666, -28.036) (134.2615, -27.9204) (133.9559, -27.8069) (133.6497, -27.6954) (133.3429, -27.5868) (133.0346, -27.4836) (132.7242, -27.3894) (132.4735, -27.3238) (132.2837, -27.2815) (132.1564, -27.2565) (132.0926, -27.2448) knots -1 -1 -1 -1 -1 -1 -0.98571429 -0.97142857 -0.95714286 -0.94285714 -0.92857143 -0.91428571 -0.9 -0.88571429 -0.87142857 -0.85714286 -0.84285714 -0.82857143 -0.81428571 -0.8 -0.78571429 -0.77142857 -0.75714286 -0.74285714 -0.72857143 -0.71428571 -0.7 -0.68571429 -0.67142857 -0.65714286 -0.64285714 -0.62857143 -0.61428571 -0.6 -0.58571429 -0.57142857 -0.55714286 -0.54285714 -0.52857143 -0.51428571 -0.5 -0.48571429 -0.47142857 -0.45714286 -0.44285714 -0.42857143 -0.41428571 -0.4 -0.38571429 -0.37142857 -0.35714286 -0.34285714 -0.32857143 -0.31428571 -0.3 -0.28571429 -0.27142857 -0.25714286 -0.24285714 -0.22857143 -0.21428571 -0.2 -0.18571429 -0.17142857 -0.15714286 -0.14285714 -0.12857143 -0.11428571 -0.1 -0.08571429 -0.07142857 -0.05714286 -0.04285714 -0.02857143 -0.01428571 0 0 0 0 0 0
  line L47 (132.0926, -27.2448) -> (127.6452, -26.4282)
  arc A95 (126.3672, -24.5983) -> (127.6452, -26.4282) centre (127.9319, -24.8668) ccw
  circle A96 centre (-8.7656, -1.4025) radius 12.7
  circle A97 centre (-8.7656, -1.4025) radius 12.7
  dimension "d20" = 25.4
  constraint concentric A0 A97
  measures "d20" diameter of A97
extrude "Extrude1'''" add sketch "Sketch2 (3)" along normal mid plane 152.4 separate body contours A96 A97 makes body 4 in component "Component'"
component "Spur Gear (24 teeth)" placed x (1, 0, 0) y (0, 1, 0) z (0, 0, 1) at (-8.7656, -1.4025, 0)
component "Spur Gear (48 teeth)" placed x (1, 0, 0) y (0, 1, 0) z (0, 0, 1) at (454.6829, 23.7432, 0)
component "Component" placed x (1, 0, 0) y (0, 1, 0) z (0, 0, 1) at (0, 0, 0)
component "Component'" placed x (1, 0, 0) y (0, 1, 0) z (0, 0, 1) at (0, 0, 0)
